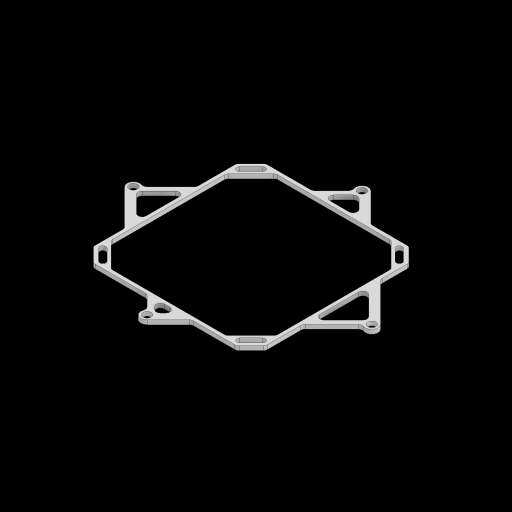
# Autodesk Inventor part: Frame
Saved by Autodesk Inventor 2023.1 (Build 271208000, 208)
## iProperties
Created: 2022-11-28
Part Number: Frame
Material: Generic
Document SubType Name: Modeling
Designer: Jose
Density: 1 g/cm^3
Appearance: Default
Author: Jose
Autodesk Inventor part; units mm, degrees
ref_plane "YZ Plane" through (0, 0, 0) normal (1, 0, 0) x (0, 1, 0)
ref_plane "XZ Plane" through (0, 0, 0) normal (0, 1, 0) x (-1, 0, 0)
ref_plane "XY Plane" through (0, 0, 0) normal (0, 0, 1) x (1, 0, 0)
sketch "Sketch1" plane through (0, 0, 0) normal (0, 1, 0) x (-1, 0, 0)
  line L0 (-41.45, 41.45) -> (41.45, 41.45) construction
  line L1 (41.45, 41.45) -> (41.45, -41.45) construction
  line L2 (41.45, -41.45) -> (-41.45, -41.45) construction
  line L3 (-41.45, -41.45) -> (-41.45, 41.45) construction
  point P0 (0, 0)
  point P1 (41.45, 0)
  point P2 (0, -41.45)
  dimension "d37" = 82.9
  dimension "d44" = 82.9
  constraints: 2 midpoint, 1 horizontal, 1 horizontal alignment, 1 vertical alignment, 2 other
  measures "d37" distance between parallel lines of L3 L1
  measures "d44" distance between parallel lines of L0 L2
sketch "Sketch2" plane through (0, 0, 0) normal (0, 1, 0) x (-1, 0, 0)
  line L0 (41.45, 41.45) -> (-41.45, -41.45) construction
  line L1 (-25.9651, -41.3786) -> (-39.6786, -27.6651)
  line L2 (-34.4504, -41.3786) -> (-41.3786, -34.4504)
  line L3 (-25.9651, -41.3786) -> (-34.4504, -41.3786)
  line L4 (-41.3786, 28.5496) -> (-41.3786, -34.4504)
  line L5 (-39.6786, -27.6651) -> (-39.6786, 28.5496)
  line L6 (-39.6786, 28.5496) -> (-41.3786, 28.5496)
  line L7 (-32.9253, -38.3747) -> (-38.3747, -32.9253) construction
  line L8 (-31.9, -37.3494) -> (-37.3494, -31.9)
  line L9 (-39.4, -33.9506) -> (-33.9506, -39.4)
  arc A0 (-33.9506, -39.4) -> (-31.9, -37.3494) centre (-32.9253, -38.3747) ccw
  arc A1 (-37.3494, -31.9) -> (-39.4, -33.9506) centre (-38.3747, -32.9253) ccw
  point P0 (41.45, -41.45)
  point P1 (-41.45, 41.45)
  point P2 (-35.65, -35.65)
  point P3 (-39.4, -31.9)
  point P4 (-31.9, -39.4)
  dimension "d51" = 6
  dimension "d52" = 5
  dimension "d54" = 1.7
  dimension "d55" = 63
  dimension "d56" = 7
  dimension "d57" = 7
  dimension "d58" = 2.9
  dimension "d60" = 5.8
  dimension "d61" = 7.5
  constraints: 22 end point, 6 point on circle, 4 tangent, 3 perpendicular, 2 centre point, 2 horizontal, 2 parallel, 1 coincident, 1 midpoint, 1 point on line, 1 vertical
  measures "d51" distance between parallel lines of L2 L1
  measures "d52" distance from line of L0.end L2
  measures "d54" distance between parallel lines of L4 L5
  measures "d55" distance of L4.start L2.end
  measures "d56" distance of L0.end L2.end
  measures "d57" distance of L0.end L2.start
  measures "d58" distance between parallel lines of L9 L8
  measures "d60" horizontal distance of L0.end point (-35.65, -35.65)
  measures "d61" horizontal distance of point (-39.4, -31.9) point (-31.9, -39.4)
extrude "Extrusion1" add sketch "Sketch2" along normal blind 2
pattern_circular "Circular Pattern1" count 4 over 360 about axis through (0, -10, 0) along (0, 1, 0) of "Extrusion1"
fillet "Fillet1" radius 2 8 edges at (-41.3786, 1, -34.4504) (-34.4504, 1, -41.3786) (34.4504, 1, -41.3786) (41.3786, 1, -34.4504) (41.3786, 1, 34.4504) (34.4504, 1, 41.3786) (-41.3786, 1, 34.4504) (-34.4504, 1, 41.3786)
fillet "Fillet2" radius 2 8 edges at (39.6786, 1, -27.6651) (27.6651, 1, -39.6786) (-39.6786, 1, -27.6651) (-27.6651, 1, -39.6786) (-27.6651, 1, 39.6786) (-39.6786, 1, 27.6651) (39.6786, 1, 27.6651) (27.6651, 1, 39.6786)
sketch "Sketch4" plane through (0, 0, 0) normal (0, 1, 0) x (-1, 0, 0)
  line L0 (33.6219, 41.3786) -> (-33.6219, 41.3786) projected
  arc A0 (2.1213, 47.8787) -> (-2.1213, 52.1213) centre (0, 50) ccw
  line L1 (-2.1213, 52.1213) -> (-12.8641, 41.3786)
  line L2 (-9.0001, 59.0001) -> (9.0001, 40.9999) construction
  line L3 (0, 49.2171) -> (0, 50.7829) construction
  line L4 (2.1213, 47.8787) -> (8.6214, 41.3786)
  line L5 (-1.0607, 47.5251) -> (5.0859, 41.3786)
  circle A1 centre (0, 50) radius 2
  line L6 (-1.0607, 47.5251) -> (-7.2072, 41.3786)
  point P0 (0, 0)
  point P1 (-14.3788, 41.3786)
  dimension "d82" = 6
  dimension "d84" = 50
  dimension "d87" = 45
  dimension "d88" = 2.5
  dimension "d89" = 4
  dimension "d93" = 4
  constraints: 12 end point, 8 point on line, 3 perpendicular, 2 centre point, 2 coincident, 2 midpoint, 2 point on circle, 1 parallel, 1 tangent, 1 vertical, 1 vertical alignment
  measures "d82" diameter of A0
  measures "d84" distance of point (0, 0) A0.centre
  measures "d87" angle of L2 L3
  measures "d88" distance between parallel lines of L5 L4
  measures "d89" diameter of A1
  measures "d93" distance between parallel lines of L1 L6
extrude "Extrusion2" add sketch "Sketch4" along normal blind 2 contours L0 L5 L6 L1 A0 L4
sketch "Sketch5" plane through (29.7715, 2, 5.1458) normal (0, 1, 0) x (0, 0, -1)
  line L0 (38.7677, 71.1501) -> (-28.4761, 71.1501)
  arc A0 (7.2671, 84.2502) -> (3.0245, 88.4929) centre (5.1458, 86.3715) ccw
  line L1 (3.0245, 88.4929) -> (-14.3183, 71.1501)
  line L2 (8.4586, 83.0587) -> (1.833, 89.6843) construction
  line L3 (5.1458, 49.2171) -> (5.1458, 123.526) construction
  line L4 (7.2671, 84.2502) -> (20.3672, 71.1501)
  line L5 (4.0851, 83.8967) -> (16.8317, 71.1501)
  circle A1 centre (5.1458, 86.3715) radius 2
  line L6 (4.0851, 83.8967) -> (-8.6614, 71.1501)
  point P0 (5.1458, 29.7715)
  point P1 (-17.4354, 71.1501)
  point P2 (5.1458, 29.7715)
  dimension "d101" = 6
  dimension "d102" = 56.6
  dimension "d100" = 45
  dimension "d99" = 2.5
  dimension "d98" = 4
  dimension "d97" = 4
  constraints: 14 end point, 8 point on line, 5 coincident, 3 perpendicular, 2 centre point, 2 midpoint, 2 point on circle, 1 parallel, 1 tangent, 1 vertical, 1 vertical alignment
  measures "d101" diameter of A0
  measures "d102" distance of point (5.146, 29.772) A0.centre
  measures "d100" angle of L2 L3
  measures "d99" distance between parallel lines of L5 L4
  measures "d98" diameter of A1
  measures "d97" distance between parallel lines of L1 L6
extrude "Extrusion3" add sketch "Sketch5" against normal blind 2 contours L0 L5 L6 L1 A0 L4
sketch "Sketch6" plane through (-4.3834, 0, 34.3718) normal (0, -1, 0) x (-1, 0, 0)
  line L0 (30.0039, 75.5981) -> (-38.0054, 75.7504)
  arc A0 (-2.2621, 85.5505) -> (-6.5047, 89.7931) centre (-4.3834, 87.6718) ccw
  line L1 (-6.5047, 89.7931) -> (-20.5865, 75.7114)
  line L2 (5.9941, 77.2942) -> (-14.761, 98.0493) construction
  line L3 (-4.3834, 49.2171) -> (-4.3834, 126.1265) construction
  line L4 (-2.2621, 85.5505) -> (7.6402, 75.6482)
  line L5 (-5.4441, 85.1969) -> (4.0967, 75.6561)
  circle A1 centre (-4.3834, 87.6718) radius 2
  line L6 (-5.4441, 85.1969) -> (-14.9423, 75.6987)
  arc A2 (30.6527, 75.1646) -> (29.2385, 75.7504) centre (29.2385, 73.7504) ccw projected
  point P0 (-4.3834, 34.3718)
  point P1 (-19.8986, 75.7098)
  point P2 (-4.3834, 34.3718)
  dimension "d110" = 6
  dimension "d111" = 53.3
  dimension "d109" = 45
  dimension "d108" = 2.5
  dimension "d107" = 4
  dimension "d106" = 4
  constraints: 14 end point, 8 point on line, 4 coincident, 3 perpendicular, 3 point on circle, 2 centre point, 2 midpoint, 1 parallel, 1 tangent, 1 vertical, 1 vertical alignment
  measures "d110" diameter of A0
  measures "d111" distance of point (-4.383, 34.372) A0.centre
  measures "d109" angle of L2 L3
  measures "d108" distance between parallel lines of L5 L4
  measures "d107" diameter of A1
  measures "d106" distance between parallel lines of L1 L6
extrude "Extrusion4" add sketch "Sketch6" against normal blind 2 contours L0 L5 L6 L1 A0 L4
sketch "Sketch7" plane through (-33.2606, 2, 0.2218) normal (0, 1, 0) x (0, 0, 1)
  line L0 (33.4001, 74.6391) -> (-33.8438, 74.6391)
  arc A0 (1.8995, 89.1393) -> (-2.3431, 93.3819) centre (-0.2218, 91.2606) ccw
  line L1 (-2.3431, 93.3819) -> (-21.0859, 74.6391)
  line L2 (7.5193, 83.5194) -> (-7.963, 99.0017) construction
  line L3 (-0.2218, 49.2171) -> (-0.2218, 133.304) construction
  line L4 (1.8995, 89.1393) -> (16.3996, 74.6391)
  line L5 (-1.2825, 88.7857) -> (12.8641, 74.6391)
  circle A1 centre (-0.2218, 91.2606) radius 2
  line L6 (-1.2825, 88.7857) -> (-15.429, 74.6391)
  point P0 (-0.2218, 33.2606)
  point P1 (-5.2716, 74.6391)
  point P2 (-0.2218, 33.2606)
  dimension "d119" = 6
  dimension "d120" = 58
  dimension "d118" = 45
  dimension "d117" = 2.5
  dimension "d116" = 4
  dimension "d115" = 4
  constraints: 14 end point, 8 point on line, 5 coincident, 3 perpendicular, 2 centre point, 2 midpoint, 2 point on circle, 1 parallel, 1 tangent, 1 vertical, 1 vertical alignment
  measures "d119" diameter of A0
  measures "d120" distance of point (-0.222, 33.261) A0.centre
  measures "d118" angle of L2 L3
  measures "d117" distance between parallel lines of L5 L4
  measures "d116" diameter of A1
  measures "d115" distance between parallel lines of L1 L6
extrude "Extrusion5" add sketch "Sketch7" against normal blind 2 contours L0 L5 L6 L1 A0 L4
fillet "Fillet4" radius 2 24 edges at (41.3786, 1, -20.8641) (55.5251, 1, -1.0607) (41.3786, 1, -15.2072) (55.8787, 1, 2.1213) (41.3786, 1, 16.6214) (41.3786, 1, 13.0859) (12.8641, 1, 41.3786) (1.0607, 1, 47.5251) (7.2072, 1, 41.3786) (-5.0859, 1, 41.3786) (-8.6214, 1, 41.3786) (-2.1213, 1, 47.8787) (-41.3786, 1, 19.4641) (-41.3786, 1, 13.8072) (-41.3786, 1, -11.6859) (-54.1251, 1, 1.0607) (-54.4787, 1, -2.1213) (-41.3786, 1, -15.2214) (-11.9214, 1, -41.3786) (-8.3859, 1, -41.3786) (10.5072, 1, -41.3786) (16.1641, 1, -41.3786) (1.0607, 1, -50.8251) (-2.1213, 1, -51.1787)
body "Solid1"
